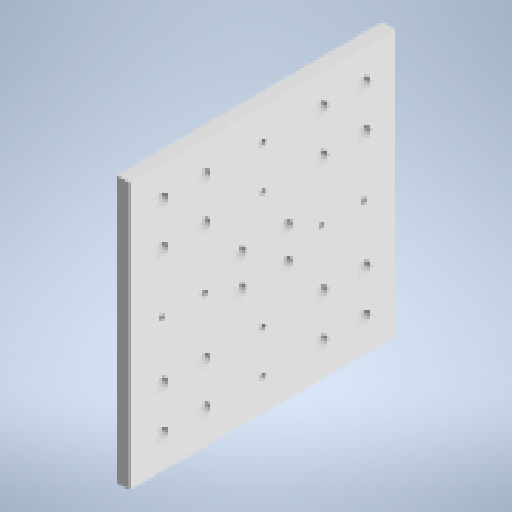
# Autodesk Inventor part: bantruot
Saved by Autodesk Inventor 2023 (Build 270158000, 158)
## iProperties
Created: 2025-04-10
Part Number: bantruot
Material: Generic
Document SubType Name: Modeling
Designer: LENOVO
Density: 1 g/cm^3
Appearance: Default
Author: LENOVO
Autodesk Inventor part; units mm, degrees
ref_plane "YZ Plane" through (0, 0, 0) normal (1, 0, 0) x (0, 1, 0)
ref_plane "XZ Plane" through (0, 0, 0) normal (0, 1, 0) x (-1, 0, 0)
ref_plane "XY Plane" through (0, 0, 0) normal (0, 0, 1) x (1, 0, 0)
sketch "Sketch1" plane through (0, 0, 0) normal (1, 0, 0) x (0, 1, 0)
  line L0 (0, 0) -> (200, 0)
  line L1 (200, 0) -> (200, -200)
  line L2 (200, -200) -> (0, -200)
  line L3 (0, -200) -> (0, 0)
  dimension "d0" = 200
  dimension "d1" = 200
  constraints: 8 end point, 2 parallel, 1 horizontal, 1 perpendicular
  measures "d0" distance of L1.end L2.end
  measures "d1" distance of L0.end L1.end
extrude "Extrusion1" add sketch "Sketch1" along normal blind 10
sketch "Sketch2" plane through (10, 0, 0) normal (1, 0, 0) x (0, 0, -1)
  circle A0 centre (24, 176) radius 2.5
  circle A1 centre (56, 176) radius 2.5
  circle A2 centre (24, 144) radius 2.5
  circle A3 centre (56, 144) radius 2.5
  line L0 (0, 200) -> (0, 0) projected
  line L1 (0, 100) -> (200, 100)
  line L2 (200, 0) -> (200, 200) projected
  line L3 (24, 176) -> (56, 176)
  line L4 (24, 176) -> (24, 144)
  line L5 (200, 200) -> (0, 200) projected
  line L6 (100, 200) -> (100, 0)
  line L7 (0, 0) -> (200, 0) projected
  circle A4 centre (176, 176) radius 2.5
  circle A5 centre (144, 176) radius 2.5
  circle A6 centre (176, 144) radius 2.5
  circle A7 centre (144, 144) radius 2.5
  line L8 (176, 176) -> (144, 176)
  line L9 (176, 176) -> (176, 144)
  circle A8 centre (24, 24) radius 2.5
  circle A9 centre (56, 24) radius 2.5
  circle A10 centre (24, 56) radius 2.5
  circle A11 centre (56, 56) radius 2.5
  line L10 (24, 24) -> (56, 24)
  line L11 (24, 24) -> (24, 56)
  line L12 (176, 24) -> (144, 24)
  line L13 (176, 24) -> (176, 56)
  circle A12 centre (144, 24) radius 2.5
  circle A13 centre (176, 56) radius 2.5
  circle A14 centre (144, 56) radius 2.5
  circle A15 centre (176, 24) radius 2.5
  circle A16 centre (82.5, 112) radius 2.5
  circle A17 centre (117.5, 112) radius 2.5
  circle A18 centre (82.5, 88) radius 2.5
  circle A19 centre (117.5, 88) radius 2.5
  point P0 (40, 176)
  point P1 (24, 160)
  point P2 (160, 176)
  point P3 (176, 160)
  point P4 (40, 24)
  point P5 (24, 40)
  point P6 (160, 24)
  point P7 (176, 40)
  dimension "d4" = 5
  dimension "d5" = 5
  dimension "d6" = 5
  dimension "d7" = 5
  dimension "d8" = 32
  dimension "d10" = 32
  dimension "d11" = 32
  dimension "d12" = 40
  dimension "d14" = 40
  dimension "d41" = 5
  dimension "d42" = 5
  dimension "d43" = 5
  dimension "d44" = 5
  dimension "d45" = 35
  dimension "d46" = 24
  dimension "d47" = 12
  dimension "d48" = 17.5
  dimension "d49" = 32
  dimension "d50" = 44
  dimension "d51" = 24
  dimension "d52" = 24
  constraints: 20 centre point, 20 end point, 18 symmetric about line, 6 midpoint, 3 horizontal alignment, 3 vertical alignment, 12 other
  measures "d4" diameter of A0
  measures "d5" diameter of A1
  measures "d6" diameter of A2
  measures "d7" diameter of A3
  measures "d8" distance of L3.end L3.start
  measures "d10" distance of A3.centre L3.end
  measures "d11" distance of A3.centre L4.end
  measures "d12" distance from line of point (40, 176) L0
  measures "d14" distance from line of L5 point (24, 160)
  measures "d41" diameter of A16
  measures "d42" diameter of A17
  measures "d43" diameter of A18
  measures "d44" diameter of A19
  measures "d45" distance of A17.centre A16.centre
  measures "d46" distance of A18.centre A16.centre
  measures "d47" distance from line of L1 A16.centre
  measures "d48" distance from line of L6 A16.centre
  measures "d49" distance of L4.end L3.start
  measures "d50" distance from line of L1 L4.end
  measures "d51" distance from line of L0 L3.start
  measures "d52" distance from line of L5 L3.start
hole "Hole1" at (10, 176, -24) at (10, 176, -56) at (10, 144, -24) at (10, 144, -56) at (10, 176, -144) at (10, 176, -176) at (10, 144, -144) at (10, 144, -176) at (10, 56, -24) at (10, 56, -56) at (10, 24, -24) at (10, 24, -56) at (10, 56, -144) at (10, 56, -176) at (10, 24, -176) at (10, 24, -144) at (10, 112, -82.5) at (10, 112, -117.5) at (10, 88, -82.5) at (10, 88, -117.5) direction (-1, 0, 0) diameter 6 end through all counterbore diameter 10 counterbore depth 5
sketch "Sketch4" plane through (10, 0, 0) normal (1, 0, 0) x (0, 0, -1)
  line L0 (200, 200) -> (0, 200) projected
  line L1 (100, 200) -> (100, 0)
  line L2 (0, 0) -> (200, 0) projected
  line L3 (0, 200) -> (0, 0) projected
  line L4 (0, 100) -> (200, 100)
  line L5 (200, 0) -> (200, 200) projected
  circle A0 centre (24, 100) radius 2.5
  circle A1 centre (56, 100) radius 2.5
  circle A2 centre (176, 100) radius 2.5
  circle A3 centre (144, 100) radius 2.5
  circle A4 centre (100, 176) radius 2.5
  circle A5 centre (100, 144) radius 2.5
  circle A6 centre (82.5, 88) radius 5 projected
  circle A7 centre (82.5, 112) radius 5 projected
  circle A8 centre (176, 24) radius 5 projected
  circle A9 centre (144, 56) radius 5 projected
  circle A10 centre (24, 24) radius 5 projected
  circle A11 centre (24, 56) radius 5 projected
  circle A12 centre (144, 144) radius 5 projected
  circle A13 centre (144, 176) radius 5 projected
  circle A14 centre (24, 144) radius 5 projected
  circle A15 centre (24, 176) radius 5 projected
  circle A16 centre (56, 176) radius 5 projected
  circle A17 centre (56, 144) radius 5 projected
  circle A18 centre (176, 176) radius 5 projected
  circle A19 centre (176, 144) radius 5 projected
  circle A20 centre (56, 56) radius 5 projected
  circle A21 centre (56, 24) radius 5 projected
  circle A22 centre (176, 56) radius 5 projected
  circle A23 centre (144, 24) radius 5 projected
  circle A24 centre (117.5, 112) radius 5 projected
  circle A25 centre (117.5, 88) radius 5 projected
  line L6 (200, 0) -> (200, 200) projected
  line L7 (200, 200) -> (0, 200) projected
  line L8 (0, 200) -> (0, 0) projected
  line L9 (0, 0) -> (200, 0) projected
  circle A26 centre (100, 24) radius 2.5
  circle A27 centre (100, 56) radius 2.5
  dimension "d53" = 5
  dimension "d54" = 5
  dimension "d55" = 32
  dimension "d56" = 24
  dimension "d57" = 5
  dimension "d58" = 5
  dimension "d59" = 32
  dimension "d60" = 24
  constraints: 8 centre point, 4 end point, 4 midpoint, 4 point on line, 4 symmetric about line, 4 other
  measures "d53" diameter of A0
  measures "d54" diameter of A1
  measures "d55" distance of A1.centre A0.centre
  measures "d56" distance from line of L3 A0.centre
  measures "d57" diameter of A4
  measures "d58" diameter of A5
  measures "d59" distance of A5.centre A4.centre
  measures "d60" distance from line of L0 A4.centre
hole "Hole2" at (10, 100, -24) at (10, 100, -56) at (10, 176, -100) at (10, 144, -100) at (10, 100, -144) at (10, 100, -176) at (10, 56, -100) at (10, 24, -100) direction (-1, 0, 0) diameter 4.134 end through all thread size "M5x0.8" class "6H" standard "ISO Metric profile"
sketch "Sketch5" plane through (0, 0, 0) normal (0, 0, 1) x (1, 0, 0)
  circle A0 centre (5, 65) radius 2.5
  line L0 (10, 200) -> (10, 0) projected
  line L1 (0, 0) -> (10, 0) projected
  dimension "d68" = 5
  dimension "d69" = 5
  dimension "d70" = 65
  constraints: 1 centre point
  measures "d68" diameter of A0
  measures "d69" distance from line of L0 A0.centre
  measures "d70" distance from line of L1 A0.centre
hole "Hole3" at (5, 65, 0) direction (0, 0, -1) diameter 4.134 depth 14.2 tip angle 118 thread size "M5x0.8" class "6H" standard "ISO Metric profile"
body "Solid1"
